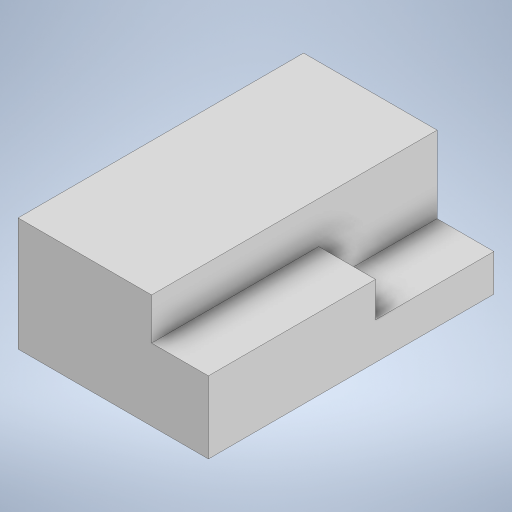
# Autodesk Inventor part: New Board
Saved by Autodesk Inventor 2024 (Build 280153000, 153)
## iProperties
Created: 2024-02-16
Part Number: New Board
Material: Generic
Document SubType Name: Modeling
Designer: CJ110
Density: 1 g/cm^3
Appearance: Default
Author: CJ110
Autodesk Inventor part; units mm, degrees
ref_plane "YZ Plane" through (0, 0, 0) normal (1, 0, 0) x (0, 1, 0)
ref_plane "XZ Plane" through (0, 0, 0) normal (0, 1, 0) x (-1, 0, 0)
ref_plane "XY Plane" through (0, 0, 0) normal (0, 0, 1) x (1, 0, 0)
sketch "Sketch1" plane through (0, 0, 0) normal (0, 1, 0) x (-1, 0, 0)
  line L0 (0, 0) -> (40.2, 0)
  line L1 (40.2, 0) -> (40.2, 60.3)
  line L2 (40.2, 60.3) -> (0, 60.3)
  line L3 (0, 60.3) -> (0, 0)
  dimension "d0" = 60.3
  dimension "d1" = 40.2
  constraints: 8 end point, 2 parallel, 1 horizontal, 1 perpendicular
  measures "d0" distance of L0.end L1.end
  measures "d1" distance of L1.end L2.end
extrude "Extrusion1" add sketch "Sketch1" along normal blind 24
sketch "Sketch2" plane through (-40.2, 0, 60.3) normal (0, 0, 1) x (1, 0, 0)
  line L0 (0, 0) -> (40.2, 0) projected
  line L1 (40.2, 0) -> (40.2, 24) projected
  line L2 (0, 24) -> (40.2, 24) projected
  line L3 (0, 0) -> (0, 24) projected
  line L4 (40.2, 24) -> (28.2, 24)
  line L5 (28.2, 24) -> (28.2, 15.2)
  line L6 (28.2, 15.2) -> (40.2, 15.2)
  line L7 (40.2, 15.2) -> (40.2, 24)
  point P0 (40.2, 0)
  point P1 (28.2, 24)
  dimension "d4" = 12
  dimension "d5" = 8.8
  constraints: 8 end point, 2 parallel, 1 horizontal, 1 perpendicular
  measures "d4" distance between parallel lines of L5 L1
  measures "d5" distance between parallel lines of L6 L2
extrude "Extrusion2" cut sketch "Sketch2" against normal through all contours L6 L5 L2 L1
sketch "Sketch3" plane through (0, 0, 60.3) normal (1, 0, 0) x (0, 0, -1)
  line L0 (60.3, 15.2) -> (0, 15.2) projected
  line L1 (0, 0) -> (0, 15.2) projected
  line L2 (0, 0) -> (60.3, 0) projected
  line L3 (60.3, 0) -> (60.3, 15.2) projected
  line L4 (60.3, 15.2) -> (35.3, 15.2)
  line L5 (35.3, 15.2) -> (35.3, 7.8)
  line L6 (35.3, 7.8) -> (60.3, 7.8)
  line L7 (60.3, 7.8) -> (60.3, 15.2)
  dimension "d8" = 25
  dimension "d9" = 7.4
  constraints: 8 end point, 2 parallel, 1 horizontal, 1 perpendicular
  measures "d8" distance between parallel lines of L3 L5
  measures "d9" distance between parallel lines of L0 L6
extrude "Extrusion3" cut sketch "Sketch3" against normal up to surface (12 mm away) contours L3 L6 L5 L0
body "Solid1"
